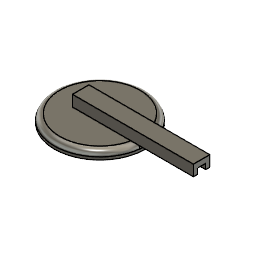
glasses_assembly_v2_d (Autodesk Fusion 360 archive; units mm, degrees)
design "nosebracket"
Autodesk Fusion 360 part; units mm, degrees
sketch "Sketch1" plane through (0, 0, 0) normal (0, 1, 0) x (1, 0, 0)
  circle A0 centre (0, 0) radius 4.75
  circle A1 centre (0, 0) radius 8.289
  dimension "d1" = 9.5
  dimension "d2" = 16.578
  constraint coincident A0.centre A1.centre
  measures "d1" diameter of A0
  measures "d2" diameter of A1
extrude "Extrude1" add sketch "Sketch1" along normal blind 1
sketch "Sketch2" plane through (0, 1, 0) normal (0, 1, 0) x (-1, 0, 0)
  circle A0 centre (0, 0) radius 4.75
  circle A1 centre (0, 0) radius 8.289
  circle A2 centre (0, 0) radius 8.289
  constraint concentric A0 A2
extrude "Extrude2" add sketch "Sketch2" along normal blind 0.5 contours A0 | A1 A2
fillet "Fillet1" radius 1 1 faces at (-2.7321, 1.5, -0.4118)
sketch "Sketch3" plane through (0, 1.5, 0) normal (0, 1, 0) x (-1, 0, 0)
  circle A0 centre (0, 0) radius 7.289
  line L0 (0, 0) -> (2, 0)
  line L1 (0.5, 1.5) -> (3.5, 1.5)
  line L2 (3.5, 1.5) -> (3.5, -1.5)
  line L3 (3.5, -1.5) -> (0.5, -1.5)
  line L4 (0.5, -1.5) -> (0.5, 1.5)
  line L5 (0.5, 1.5) -> (3.5, -1.5) construction
  line L6 (3.5, 1.5) -> (0.5, -1.5) construction
  line L7 (0, 0) -> (0, 1)
  line L8 (0, 1) -> (-8.289, 1)
  line L9 (-8.289, 1) -> (-8.289, -1)
  line L10 (-8.289, -1) -> (0, -1)
  line L11 (0, -1) -> (0, 1)
  point P0 (2, 0)
  dimension "d10" = 2
  dimension "d13" = 3
  dimension "d14" = 3
  dimension "d19" = 1
  dimension "d20" = 8.289
  dimension "d21" = 2
  constraint coincident A0.centre L0.start
  constraint horizontal L0
  constraint horizontal L1
  constraint perpendicular L1 L2
  constraint parallel L1 L3
  constraint parallel L2 L4
  constraint coincident L5 P0
  constraint coincident L6 P0
  constraint coincident P0 L0.end
  constraint vertical L7
  constraint horizontal L8
  constraint vertical L9
  constraint horizontal L10
  constraint vertical L11
  measures "d10" distance of A0.centre P0
  measures "d13" distance of L2.end L3.end
  measures "d14" distance of L1.end L2.end
  measures "d19" distance of A0.centre L7.end
  measures "d20" distance of L7.end L8.end
  measures "d21" distance of L7.end L10.end
extrude "Extrude4" add sketch "Sketch3" along normal blind 2 contours L1 L2 L3 L4
extrude "Extrude5" cut sketch "Sketch3" against normal blind 1 contours A0 L7 L8 L10 L11 | A0 L8 L9 L10 picked at (-2.4067, -0.6667)
extrude "Extrude6" add 1 faces at (-0.5, 2.8333, 0.5) along direction (1, 0, 0) blind 19
sketch "Sketch4" plane through (18.5, 0, 0) normal (1, 0, 0) x (0, 0, -1)
  line L0 (-1.5, 1.5) -> (1.5, 1.5)
  line L1 (1.5, 1.5) -> (1.5, 3.5)
  line L2 (1.5, 3.5) -> (-1.5, 3.5)
  line L3 (-1.5, 3.5) -> (-1.5, 1.5)
  line L4 (-1.5, 1.5) -> (-0.75, 1.5)
  line L5 (-0.75, 1.5) -> (0.75, 1.5)
  line L6 (0.75, 1.5) -> (0.75, 2.5)
  line L7 (0.75, 2.5) -> (-0.75, 2.5)
  line L8 (-0.75, 2.5) -> (-0.75, 1.5)
  dimension "d26" = 0.75
  dimension "d27" = 1.5
  dimension "d28" = 1
  constraint horizontal L4
  constraint coincident L0.start L3.end
  constraint horizontal L5
  constraint vertical L6
  constraint horizontal L7
  constraint vertical L8
  measures "d26" distance of L0.start L4.end
  measures "d27" distance of L4.end L5.end
  measures "d28" distance of L4.end L7.end
extrude "Extrude7" cut sketch "Sketch4" against normal blind 18.5 contours L0 L5 L6 L7 L8

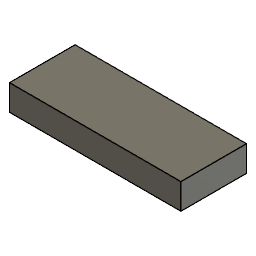
design "battery"
Autodesk Fusion 360 part; units mm, degrees
sketch "Sketch1" plane through (0, 0, 0) normal (0, 1, 0) x (1, 0, 0)
  line L0 (0, 0) -> (30, 0)
  line L1 (30, 0) -> (30, -11.5)
  line L2 (30, -11.5) -> (0, -11.5)
  line L3 (0, -11.5) -> (0, 0)
  dimension "d1" = 30
  dimension "d2" = 11.5
  constraint horizontal L0
  constraint vertical L1
  constraint horizontal L2
  constraint vertical L3
  constraint coincident L0.start L3.end
  measures "d1" distance of L0.start L0.end
  measures "d2" distance of L0.start L2.end
extrude "Extrude1" add sketch "Sketch1" along normal blind 4.5

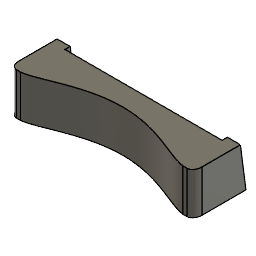
design "bridge_pad_c"
Autodesk Fusion 360 part; units mm, degrees
sketch "Sketch1" plane through (0, 0, 0) normal (0, 1, 0) x (1, 0, 0)
  line L0 (0, 0) -> (17.5, 0)
  line L1 (17.5, 0) -> (17.5, 3)
  line L2 (17.5, 3) -> (0, 3)
  line L3 (0, 3) -> (0, 0)
  line L4 (0, 0) -> (1, 0)
  line L5 (17.5, 0) -> (16.5, 0)
  line L6 (0, 3) -> (8.75, 3)
  line L7 (0, 0) -> (0, 1)
  line L8 (17.5, 0) -> (17.5, 1)
  line L9 (8.75, 3) -> (8.75, 2)
  spline S0 degree 5 poles (0, 1) (-0.0052, 0.8576) (0.0051, 0.5979) (0.0824, 0.284) (0.3098, 0.0171) (0.8015, -0.0688) (1.4966, 0.0725) (2.3822, 0.3921) (3.4374, 0.8195) (4.6351, 1.2741) (5.9435, 1.6748) (7.3276, 1.9503) (8.75, 2.049) (10.1724, 1.9503) (11.5565, 1.6748) (12.8649, 1.2741) (14.0626, 0.8195) (15.1178, 0.3921) (16.0034, 0.0725) (16.6985, -0.0688) (17.1902, 0.0171) (17.4176, 0.284) (17.4949, 0.5979) (17.5052, 0.8576) (17.5, 1) knots 0 0 0 0 0 0 0.05 0.1 0.15 0.2 0.25 0.3 0.35 0.4 0.45 0.5 0.55 0.6 0.65 0.7 0.75 0.8 0.85 0.9 0.95 1 1 1 1 1 1
  line L10 (17.5, 3) -> (0, 3)
  line L11 (0, 3) -> (0, 4.5)
  line L12 (0, 4.5) -> (17.5, 4.5)
  line L13 (17.5, 4.5) -> (17.5, 3)
  dimension "d1" = 17.5
  dimension "d2" = 3
  dimension "d3" = 1
  dimension "d4" = 1
  dimension "d5" = 8.75
  dimension "d6" = 1
  dimension "d7" = 1
  dimension "d8" = 1
  dimension "d23" = 17.5
  dimension "d24" = 1.5
  constraint horizontal L0
  constraint vertical L1
  constraint horizontal L2
  constraint vertical L3
  constraint coincident L0.start L3.end
  constraint perpendicular L3 L4
  constraint perpendicular L1 L5
  constraint perpendicular L3 L6
  constraint perpendicular L0 L7
  constraint perpendicular L0 L8
  constraint perpendicular L2 L9
  constraint horizontal L10
  constraint vertical L11
  constraint horizontal L12
  constraint vertical L13
  measures "d1" distance of L0.start L0.end
  measures "d2" distance of L0.start L2.end
  measures "d3" distance of L0.start L4.end
  measures "d4" distance of L0.end L5.end
  measures "d5" distance of L2.end L6.end
  measures "d6" distance of L0.start L7.end
  measures "d7" distance of L0.end L8.end
  measures "d8" distance of L6.end L9.end
  measures "d23" distance of L1.end L2.end
  measures "d24" distance of L1.end L12.end
extrude "Extrude1" add sketch "Sketch1" along normal blind 4 contours L0 L2 L3 L4 L6 L9 S0 L10 | L0 L1 L2 L5 L9 S0 L10 | L2 L6 L10 L11 L12 L13
draft "Draft1" angle 7.5 neutral plane through (0, 4, 0) pull (0, 1, 0) 1 faces at (5.8333, 2.6667, -4.5)
sketch "Sketch3" plane through (0, 0.6505, -4.941) normal (0, 0.130526, -0.991445) x (-1, 0, 0)
  line L0 (-17.5, -0.6561) -> (0, -0.6561)
  line L1 (0, -0.6561) -> (0, 3.3784)
  line L2 (0, 3.3784) -> (-17.5, 3.3784)
  line L3 (-17.5, 3.3784) -> (-17.5, -0.6561)
  line L4 (-17.5, 3.3784) -> (-16.25, 3.3784)
  line L5 (-16.25, 3.3784) -> (-16.25, 2.1284)
  line L6 (-16.25, 2.1284) -> (-17.5, 2.1284)
  line L7 (-17.5, 2.1284) -> (-17.5, 3.3784)
  line L8 (-16.25, 2.1284) -> (-1.25, 2.1284)
  line L9 (-1.25, 2.1284) -> (-1.25, -0.6561)
  line L10 (-1.25, -0.6561) -> (-16.25, -0.6561)
  line L11 (-16.25, -0.6561) -> (-16.25, 2.1284)
  line L12 (-1.25, 2.1284) -> (0, 2.1284)
  line L13 (-1.25, 2.1284) -> (-1.25, 3.3784)
  line L14 (-16.25, 3.3784) -> (-1.25, 3.3784)
  line L15 (-1.25, 3.3784) -> (-1.25, 4.3784)
  line L16 (-1.25, 4.3784) -> (-16.25, 4.3784)
  line L17 (-16.25, 4.3784) -> (-16.25, 3.3784)
  dimension "d25" = 1.25
  dimension "d26" = 1.25
  dimension "d34" = 1
  constraint horizontal L4
  constraint vertical L5
  constraint horizontal L6
  constraint vertical L7
  constraint coincident L2.end L3.start
  constraint horizontal L8
  constraint vertical L9
  constraint horizontal L10
  constraint vertical L11
  constraint coincident L0 L10.end
  constraint coincident L1 L12.end
  constraint perpendicular L1 L12
  constraint equal L6 L12
  constraint coincident L2 L13.end
  constraint perpendicular L2 L13
  constraint horizontal L14
  constraint vertical L15
  constraint horizontal L16
  constraint vertical L17
  constraint coincident L13.end L14.end
  measures "d25" distance of L2.end L4.end
  measures "d26" distance of L2.end L6.end
  measures "d34" distance of L4.end L16.end
extrude "Extrude3" cut sketch "Sketch3" against normal blind 1.5 contours L0 L8 L9 L10 L11
extrude "Extrude4" cut sketch "Sketch3" against normal blind 0.5 contours L2 L5 L8 L13 L14 | L2 L14 L15 L16 L17
fillet "Fillet1" [suppressed]
